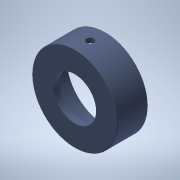
# Autodesk Inventor part: Rolamento_Inferior_Base
Saved by Autodesk Inventor 2022 (Build 260153000, 153)
## iProperties
Created: 2016-03-03
Part Number: Rolamento_Inferior_Base
Material: Genérico
Document SubType Name: Modeling
Designer: Everton
Density: 1 g/cm^3
Appearance: Padrão
Author: Everton
Autodesk Inventor part; units mm, degrees
ref_plane "YZ Plane" through (0, 0, 0) normal (1, 0, 0) x (0, 1, 0)
ref_plane "XZ Plane" through (0, 0, 0) normal (0, 1, 0) x (-1, 0, 0)
ref_plane "XY Plane" through (0, 0, 0) normal (0, 0, 1) x (1, 0, 0)
sketch "Sketch1" plane through (0, 0, 0) normal (0, 1, 0) x (-1, 0, 0)
  circle A0 centre (7.858, -16.0999) radius 70
  circle A1 centre (7.858, -16.0999) radius 35
  point P0 (0, 0)
  dimension "d0" = 140
  dimension "d1" = 70
  constraints: 2 centre point, 1 coincident
  measures "d0" diameter of A0
  measures "d1" diameter of A1
extrude "Extrusion1" add sketch "Sketch1" along normal blind 10
sketch "Sketch2" plane through (-7.858, 10, -16.0999) normal (0, 1, 0) x (1, 0, 0)
  circle A0 centre (0, 0) radius 70
  circle A1 centre (0, 0) radius 62.5
  line L0 (0, 0) -> (69.5, 0)
  line L1 (69.5, 0) -> (69.5, 27.6538)
  line L2 (69.5, 27.6538) -> (69.5, -15.3132)
  line L3 (0, 0) -> (-69.5, 0)
  line L4 (-69.5, 0) -> (-69.5, 45.4592)
  point P0 (7.858, -16.0999)
  dimension "d4" = 125
  dimension "d14" = 140
  dimension "d19" = 69.5
  dimension "d20" = 69.5
  constraints: 10 end point, 2 centre point, 2 horizontal, 2 perpendicular, 1 coincident, 1 point on line
  measures "d4" diameter of A1
  measures "d14" diameter of A0
  measures "d19" distance of L0.start L0.end
  measures "d20" distance of L0.start L3.end
extrude "Extrusion2" add sketch "Sketch2" along normal blind 40 contours A0 L2 L1 | L1 L0 A1 L3 L4 A0 | A0 L4 L3 A1 L0 L2
sketch "Sketch3" plane through (-7.858, 10, -16.0999) normal (0, 1, 0) x (1, 0, 0)
  circle A0 centre (0, 0) radius 42.5
  circle A1 centre (0, 0) radius 60.5
  point P0 (7.858, -16.0999)
  dimension "d7" = 85
  constraints: 2 centre point, 1 coincident
  measures "d7" diameter of A0
extrude "Extrusion3" cut sketch "Sketch3" against normal blind 3
fillet "Fillet1" radius 3 1 edges at (-68.358, 7, -16.0999)
fillet "Fillet2" radius 3 1 edges at (-50.358, 7, -16.0999)
fillet "Fillet3" radius 1 2 edges at (-77.858, 50, -16.0999) (-70.358, 50, -16.0999)
fillet "Fillet4" radius 1 1 edges at (62.142, 0, -16.0999)
sketch "Sketch4" plane through (0, 0, 0) normal (0, 1, 0) x (-1, 0, 0)
  point P0 (0, 0)
sketch "Sketch5" plane through (0, 0, 0) normal (0, 0, 1) x (1, 0, 0)
  line L0 (-77.858, 1) -> (62.142, 1) projected
  line L1 (62.1388, 1) -> (-77.858, 49)
  line L2 (62.142, 49) -> (-77.858, 49) projected
  circle A0 centre (-7.8596, 25) radius 6
  point P0 (0, 0)
  dimension "d15" = 12
  constraints: 3 end point, 1 centre point, 1 midpoint, 1 point on line
  measures "d15" diameter of A0
extrude "Extrusion4" cut sketch "Sketch5" along normal mid plane 300
body "Solid1"
